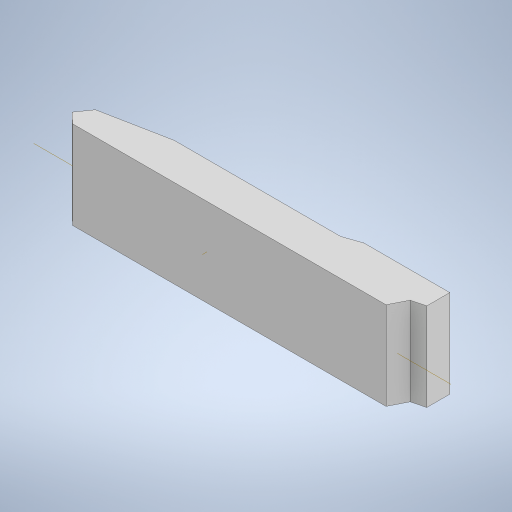
# Autodesk Inventor part: Friend_hull_collision
Saved by Autodesk Inventor 2024 (Build 280153000, 153)
## iProperties
Created: 2026-05-23
Part Number: Friend_hull_collision
Material: Generic
Document SubType Name: Modeling
Designer: warny
Density: 1 g/cm^3
Appearance: Default
Author: warny
Autodesk Inventor part; units mm, degrees
ref_plane "YZ Plane" through (0, 0, 0) normal (1, 0, 0) x (0, 1, 0)
ref_plane "XZ Plane" through (0, 0, 0) normal (0, 1, 0) x (-1, 0, 0)
ref_plane "XY Plane" through (0, 0, 0) normal (0, 0, 1) x (1, 0, 0)
sketch "Sketch1" plane through (0, 0, 0) normal (0, 1, 0) x (-1, 0, 0)
  line L0 (364.2, 20.66) -> (392.2, -5.97)
  line L1 (392.2, -5.97) -> (366, -43.36)
  line L2 (366, -43.36) -> (187.3, -78.36)
  line L3 (187.3, -78.36) -> (-264.9, -78.36)
  line L4 (-264.9, -78.36) -> (-311.9, -94.56)
  line L5 (-311.9, -94.56) -> (-544.9, -94.56)
  line L6 (-544.9, -94.56) -> (-544.9, -32.16)
  line L7 (-544.9, -32.16) -> (-508.9, -22.77)
  line L8 (-508.9, -22.77) -> (-486.9, 20.66)
  line L9 (364.2, 20.66) -> (-486.9, 20.66)
  point P0 (0, 0)
  dimension "d0" = 20.66
  dimension "d1" = 5.97
  dimension "d2" = 43.36
  dimension "d3" = 78.36
  dimension "d4" = 78.36
  dimension "d5" = 94.56
  dimension "d6" = 94.56
  dimension "d7" = 32.16
  dimension "d8" = 22.77
  dimension "d9" = 20.66
  dimension "d10" = 364.2
  dimension "d11" = 392.2
  dimension "d12" = 366
  dimension "d13" = 187.3
  dimension "d14" = 264.9
  dimension "d15" = 311.9
  dimension "d16" = 544.9
  dimension "d17" = 544.9
  dimension "d18" = 508.9
  dimension "d19" = 486.9
  constraints: 20 end point
  measures "d0" vertical distance of L0.start point (0, 0)
  measures "d1" vertical distance of L0.end point (0, 0)
  measures "d2" vertical distance of L1.end point (0, 0)
  measures "d3" vertical distance of point (0, 0) L2.end
  measures "d4" vertical distance of point (0, 0) L3.end
  measures "d5" vertical distance of point (0, 0) L4.end
  measures "d6" vertical distance of point (0, 0) L5.end
  measures "d7" vertical distance of point (0, 0) L6.end
  measures "d8" vertical distance of point (0, 0) L7.end
  measures "d9" vertical distance of L8.end point (0, 0)
  measures "d10" horizontal distance of L0.start point (0, 0)
  measures "d11" horizontal distance of point (0, 0) L0.end
  measures "d12" horizontal distance of point (0, 0) L1.end
  measures "d13" horizontal distance of point (0, 0) L2.end
  measures "d14" horizontal distance of point (0, 0) L3.end
  measures "d15" horizontal distance of point (0, 0) L4.end
  measures "d16" horizontal distance of point (0, 0) L5.end
  measures "d17" horizontal distance of point (0, 0) L6.end
  measures "d18" horizontal distance of point (0, 0) L7.end
  measures "d19" horizontal distance of point (0, 0) L8.end
extrude "Extrusion1" add sketch "Sketch1" along normal mid plane 238.9
body "Solid1"
